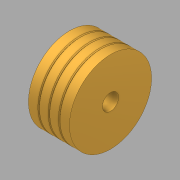
# Autodesk Inventor part: Piston
Saved by Autodesk Inventor 2020 (Build 240168000, 168)
## iProperties
Created: 2019-11-25
Part Number: Piston
Material: Latón, amarillo claro
Document SubType Name: Modeling
Designer: Gerardo Naranjo
Engineer: Gerardo Naranjo
Density: 8.47 g/cm^3
Appearance: Latón - Satinado
Title: Piston
Author: Gerardo Naranjo
Autodesk Inventor part; units mm, degrees
ref_plane "YZ Plane" through (0, 0, 0) normal (1, 0, 0) x (0, 1, 0)
ref_plane "XZ Plane" through (0, 0, 0) normal (0, 1, 0) x (-1, 0, 0)
ref_plane "XY Plane" through (0, 0, 0) normal (0, 0, 1) x (1, 0, 0)
sketch "Boceto1" plane through (0, 0, 0) normal (0, 0, 1) x (1, 0, 0)
  line L0 (0, 0) -> (-6.35, 0)
  line L1 (-6.35, 0) -> (-6.35, 6.35)
  line L2 (0, 6.35) -> (0, 0)
  line L3 (-4.7625, 6.223) -> (-4.6355, 6.35)
  line L4 (-4.7625, 6.223) -> (-4.5829, 6.223) construction
  line L5 (-4.7625, 6.223) -> (-4.8895, 6.35)
  line L6 (-4.7625, 6.223) -> (-4.5829, 6.223) construction
  line L7 (-3.175, 6.223) -> (-3.048, 6.35)
  line L8 (-3.175, 6.223) -> (-2.9954, 6.223) construction
  line L9 (-3.175, 6.223) -> (-3.302, 6.35)
  line L10 (-3.175, 6.223) -> (-2.9954, 6.223) construction
  line L11 (-1.5875, 6.223) -> (-1.4605, 6.35)
  line L12 (-1.5875, 6.223) -> (-1.4079, 6.223) construction
  line L13 (-1.5875, 6.223) -> (-1.7145, 6.35)
  line L14 (-1.5875, 6.223) -> (-1.4079, 6.223) construction
  line L15 (-6.35, 6.35) -> (-4.8895, 6.35)
  line L16 (-4.6355, 6.35) -> (-3.302, 6.35)
  line L17 (-3.048, 6.35) -> (-1.7145, 6.35)
  line L18 (-1.4605, 6.35) -> (0, 6.35)
  dimension "d0" = 6.35
  dimension "d1" = 6.35
  dimension "d3" = 1.5875
  dimension "d6" = 1.5875
  dimension "d7" = 1.5875
  dimension "d20" = 0.127
  constraints: 38 end point, 7 horizontal, 6 equal length, 5 parallel, 1 perpendicular
  measures "d0" distance of L1.end L2.start
  measures "d1" distance of L0.end L1.end
  measures "d3" distance from line of L1 L3.start
  measures "d6" distance of L3.start L7.start
  measures "d7" distance of L7.start L11.start
  measures "d20" distance between parallel lines of L12 L18
revolve "Revolución1" add sketch "Boceto1" angle 360 about axis through (0, 0, 0) along (-1, 0, 0)
sketch "Boceto2" plane through (0, 0, 0) normal (1, 0, 0) x (0, 0, -1)
  point P0 (0, 0)
  point P1 (0, 0)
  constraints: 1 coincident
hole "Agujero1" at (0, 0, 0) direction (-1, 0, 0) diameter 1.9406 end through all counterbore diameter 2.5146 counterbore depth 3.175 thread size "3-48 UNC" class "2B" standard "ANSI Unified Screw Threads"
equation "\"d7\" = d6"
